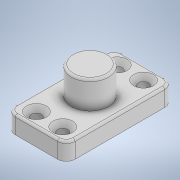
# Autodesk Inventor part: LegPin_v1
Saved by Autodesk Inventor 2020.3 (Build 243373000, 373)
## iProperties
Created: 2021-02-21
Part Number: LegPin_v1
Material: Generic
Document SubType Name: Modeling
Designer: sanyi
Density: 1 g/cm^3
Appearance: Default
Author: sanyi
Autodesk Inventor part; units mm, degrees
ref_plane "YZ Plane" through (0, 0, 0) normal (1, 0, 0) x (0, 1, 0)
ref_plane "XZ Plane" through (0, 0, 0) normal (0, 1, 0) x (-1, 0, 0)
ref_plane "XY Plane" through (0, 0, 0) normal (0, 0, 1) x (1, 0, 0)
sketch "Sketch1" plane through (0, 0, 0) normal (0, 1, 0) x (-1, 0, 0)
  line L0 (0, -21.955) -> (0, -12.2) construction
  line L1 (13.6, -21.955) -> (13.6, -12.2) construction
  line L2 (-11, -20.9069) -> (-11, 21.1673) construction
  line L3 (16.0254, 0) -> (-21.0399, 0) construction
  line L4 (13.6, -6.2) -> (0, -6.2)
  line L5 (13.6, 6.2) -> (0, 6.2)
  line L6 (6.8, -14.862) -> (6.8, 12.9569) construction
  line L7 (13.6, -6.2) -> (13.6, 6.2)
  line L8 (13.6, 6.2) -> (13.6, 12.2)
  line L9 (0, -6.2) -> (0, 6.2)
  line L10 (0, 6.2) -> (0, 12.2)
  line L11 (13.6, -12.2) -> (0, -12.2)
  line L12 (13.6, 12.2) -> (0, 12.2)
  line L13 (13.6, -12.2) -> (13.6, -6.2)
  line L14 (0, -12.2) -> (0, -6.2)
  line L15 (13.6, 12.2) -> (13.6, 20.1192) construction
  line L16 (0, 12.2) -> (0, 20.7166) construction
  line L17 (9.8, -9.2) -> (3.8, -9.2) construction
  line L18 (3.8, -9.2) -> (3.8, 9.2) construction
  line L19 (3.8, 9.2) -> (9.8, 9.2) construction
  line L20 (9.8, 9.2) -> (9.8, -9.2) construction
  circle A0 centre (6.8, 0) radius 4.25
  point P0 (0, 0)
  dimension "d0" = 24.6
  dimension "d1" = 12.4
  dimension "d2" = 6
  dimension "d4" = 6
  dimension "d17" = 8.5
  dimension "d21" = 6.8
  constraints: 42 end point, 12 perpendicular, 12 vertical, 6 point on line, 2 parallel, 1 centre point, 1 coincident, 1 horizontal, 1 midpoint, 6 other
  measures "d0" distance between parallel lines of L2 L1
  measures "d1" distance between parallel lines of L5 L4
  measures "d2" distance between parallel lines of L4 L11
  measures "d4" distance between parallel lines of L18 L20
  measures "d17" diameter of A0
  measures "d21" distance between parallel lines of L7 L6
extrude "Extrusion1" add sketch "Sketch1" along normal blind 4 contours L13 L11 L14 L4 | L5 L10 L12 L8
extrude "Extrusion2" add sketch "Sketch1" along normal blind 4 contours L4 L9 L5 L7 | A0
fillet "Fillet1" radius 2 4 edges at (0, 2, 12.2) (-13.6, 2, 12.2) (-13.6, 2, -12.2) (0, 2, -12.2)
extrude "Extrusion3" add sketch "Sketch1" along normal blind 10.3 contours A0
fillet "Fillet2" radius 0.5 7 edges at (-2.55, 10.3, 0) (-0.5858, 4, -11.6142) (-6.8, 4, -12.2) (-13.0142, 4, -11.6142) (-0.5858, 4, 11.6142) (-6.8, 4, 12.2) (-13.0142, 4, 11.6142)
sketch "Sketch3" plane through (0, 4, 0) normal (0, 1, 0) x (1, 0, 0)
  point P0 (0, 0)
  point P1 (-9.8, -9.2)
  point P2 (-3.8, -9.2)
  point P3 (-9.8, 9.2)
  point P4 (-3.8, 9.2)
hole "Hole2" at (-9.8, 4, 9.2) at (-3.8, 4, 9.2) at (-9.8, 4, -9.2) at (-3.8, 4, -9.2) direction (0, -1, 0) diameter 2.3 depth 6.5 countersink diameter 4.5 countersink angle 90
body "Solid1"
